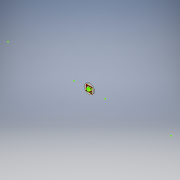
# Autodesk Inventor part: cmc
Saved by Autodesk Inventor 2018 (Build 220112000, 112)
## iProperties
Created: 2019-05-16
Part Number: cmc
Material: Generic
Document SubType Name: Modeling
Designer: F8PLTW
Density: 1 g/cm^3
Appearance: Default
Author: F8PLTW
Autodesk Inventor part; units mm, degrees
ref_plane "YZ Plane" through (0, 0, 0) normal (1, 0, 0) x (0, 1, 0)
ref_plane "XZ Plane" through (0, 0, 0) normal (0, 1, 0) x (-1, 0, 0)
ref_plane "XY Plane" through (0, 0, 0) normal (0, 0, 1) x (1, 0, 0)
sketch "Sketch1" plane through (0, 0, 0) normal (0, 0, 1) x (1, 0, 0)
  circle A0 centre (-5.1147, 3.191) radius 25.4
  point P0 (0, 0)
  dimension "d0" = 50.8
  constraints: 1 centre point
  measures "d0" diameter of A0
extrude "Extrusion1" add sketch "Sketch1" along normal blind 5.08
sketch "Sketch2" plane through (-5.1147, 3.191, 5.08) normal (0, 0, 1) x (1, 0, 0)
  point P0 (5.1147, -3.191)
sketch "Sketch3" plane through (-5.1147, 3.191, 5.08) normal (0, 0, 1) x (1, 0, 0)
  line L0 (-17.3802, 16.9544) -> (17.3231, 16.9544) construction
  line L1 (17.3231, 16.9544) -> (17.3231, -17.7488) construction
  line L2 (17.3231, -17.7488) -> (-17.3802, -17.7488) construction
  line L3 (-17.3802, -17.7488) -> (-17.3802, 16.9544) construction
  arc A0 (-5.1701, 4.4508) -> (-5.2412, 10.8446) centre (-436.8317, 2.8519) ccw
  arc A1 (2.3366, 5.7059) -> (-5.2412, 10.8446) centre (-5.4855, 2.3277) ccw
  arc A2 (2.6208, 0.6375) -> (2.3366, 5.7059) centre (-81.7267, -1.5497) ccw
  arc A3 (2.6208, 0.6375) -> (3.2602, 0.6382) centre (2.9405, 0.6457) ccw
  line L4 (2.9405, 0.6457) -> (2.9405, 3.593) construction
  arc A4 (11.1221, 10.8446) -> (11.0511, 4.4508) centre (442.7126, 2.8519) ccw
  arc A5 (11.1221, 10.8446) -> (3.5443, 5.7059) centre (11.3664, 2.3277) ccw
  arc A6 (3.5443, 5.7059) -> (3.2601, 0.6375) centre (87.6077, -1.5497) ccw
  line L5 (11.0511, 4.4508) -> (11.0511, 1.2529)
  line L6 (11.0511, 1.2529) -> (11.0121, -0.0442)
  arc A7 (11.0121, -0.0442) -> (3.3261, -4.5311) centre (11.8783, -10.3545) ccw
  line L7 (3.3261, -2.2752) -> (3.3261, -4.5311)
  arc A8 (3.3261, -2.2752) -> (2.6174, -2.2752) centre (2.9718, -2.4577) ccw
  line L8 (2.6174, -2.2752) -> (2.5501, -5.5702)
  arc A9 (0.0073, 1.8237) -> (-0.7068, -11.2689) centre (-5.3235, -4.4513) ccw
  arc A10 (-0.7068, -11.2689) -> (2.5501, -5.5702) centre (-8.8247, -2.8493) ccw
  arc A11 (0.32, 2.1194) -> (-5.1701, 4.4508) centre (-5.4429, -3.8214) ccw
  arc A12 (0.0073, 1.8237) -> (0.32, 2.1194) centre (0.1474, 1.9887) ccw
  arc A13 (-6.5958, 3.1698) -> (-6.2865, -12.2636) centre (1.6439, -4.3849) ccw
  arc A14 (-7.8328, 2.8478) -> (-7.2263, -12.4621) centre (-0.915, -4.5451) ccw
  line L9 (-7.8328, 2.8478) -> (-7.2263, 3.5596)
  line L10 (-6.2865, -12.2636) -> (-6.2865, -9.5112)
  line L11 (-6.2865, -9.5112) -> (-8.2902, -9.5112)
  line L12 (-8.7331, -8.5422) -> (-6.2865, -8.5422)
  line L13 (-6.2865, -8.5422) -> (-6.5958, -5.3834)
  line L14 (-6.5958, -5.3834) -> (-9.4902, -5.3834)
  line L15 (-9.5327, -4.161) -> (-6.5019, -4.252)
  line L16 (-6.5019, -4.252) -> (-6.5958, -0.9205)
  line L17 (-6.5958, -0.9205) -> (-9.0065, -0.9885)
  point P0 (5.1147, -3.191)
  constraints: 37 point on circle, 28 end point, 15 centre point, 7 symmetric about line, 4 vertical, 2 parallel, 2 perpendicular, 2 tangent, 1 point on line, 5 other
body "Solid1"
